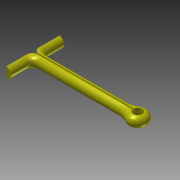
# Autodesk Inventor part: 砂轮架固定销螺丝挡销
Saved by Autodesk Inventor 2015 (Build 190159000, 159)
## iProperties
Created: 2017-05-17
Part Number: 砂轮架固定销螺丝挡销
Material: 常规
Document SubType Name: Modeling
Designer: Administrator
Density: 1 g/cm^3
Appearance: 黄色
Author: Administrator
Autodesk Inventor part; units mm, degrees
ref_plane "YZ Plane" through (0, 0, 0) normal (1, 0, 0) x (0, 1, 0)
ref_plane "XZ Plane" through (0, 0, 0) normal (0, 1, 0) x (-1, 0, 0)
ref_plane "XY Plane" through (0, 0, 0) normal (0, 0, 1) x (1, 0, 0)
sketch "草图1" plane through (0, 0, 0) normal (0, 0, 1) x (1, 0, 0)
  arc A0 (-1.436141, -1) -> (-1.436141, 1) centre (0, 0) ccw
  line L0 (0, 0) -> (5.186385, 0)
  line L1 (-1.436141, 1) -> (-18.839454, 1)
  line L2 (-1.436141, -1) -> (-18.839454, -1)
  arc A1 (-2.839454, 1) -> (-0.864182, 1.521739) centre (-2.839454, 5) ccw
  arc A2 (-0.864182, -1.521739) -> (-2.839454, -1) centre (-2.839454, -5) ccw
  line L3 (-18.839454, 1) -> (-18.839454, 5)
  line L4 (-18.839454, -1) -> (-18.839454, -5)
  line L5 (-18.839454, 5) -> (-19.739454, 5)
  line L6 (-19.739454, 5) -> (-19.739454, 0.1)
  line L7 (-19.739454, 0.1) -> (-0.844097, 0.1)
  arc A3 (-0.844097, -0.1) -> (-0.844097, 0.1) centre (0, 0) ccw
  line L8 (-0.844097, -0.1) -> (-19.739454, -0.1)
  line L9 (-19.739454, -0.1) -> (-19.739454, -5)
  line L10 (-18.839454, -5) -> (-19.739454, -5)
  dimension "d0" = 5.18639
  dimension "d1" = 1.75
  dimension "d4" = 2
  dimension "d5" = 4
  dimension "d6" = 4
  dimension "d7" = 4
  dimension "d8" = 16
  dimension "d9" = 0.9
  dimension "d10" = 4.9
  dimension "d11" = 4.9
  dimension "d12" = 0.85
  constraints: 22 end point, 10 point on circle, 4 centre point, 4 horizontal, 4 tangent, 3 parallel, 3 perpendicular, 3 point on line, 2 vertical, 1 coincident, 1 concentric, 1 symmetric about line, 1 other
  measures "d0" distance of L0.start L0.end
  measures "d1" radius of A0
  measures "d4" distance between parallel lines of L2 L1
  measures "d5" radius of A1
  measures "d6" distance of L1.end L3.end
  measures "d7" distance of L2.end L4.end
  measures "d8" distance from line of L3 A1.centre
  measures "d9" distance of L3.end L5.end
  measures "d10" distance of L5.end L6.end
  measures "d11" distance of L8.end L9.end
  measures "d12" radius of A3
extrude "拉伸1" add sketch "草图1" along normal blind 2
fillet "圆角1" radius 1 4 edges at (-18.8395, 1, 1) (-18.8395, -1, 1) (-19.7395, 0.1, 1) (-19.7395, -0.1, 1)
fillet "圆角2" radius 1 18 edges at (-1.8179, -1.1326, 2) (1.75, 0, 2) (-1.8179, 1.1326, 2) (-10.3395, 1, 2) (-18.5466, 1.2929, 2) (-18.8395, 3.5, 2) (-18.5466, -1.2929, 2) (-18.8395, -3.5, 2) (-10.3395, -1, 2) (-1.8179, -1.1326, 0) (1.75, 0, 0) (-1.8179, 1.1326, 0) (-10.3395, 1, 0) (-18.5466, 1.2929, 0) (-18.8395, 3.5, 0) (-18.5466, -1.2929, 0) (-18.8395, -3.5, 0) (-10.3395, -1, 0)
